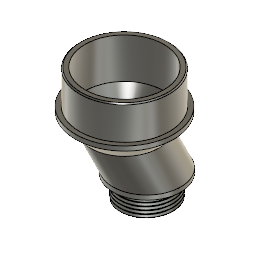
RobinairExhaustFilterAdapter (Autodesk Fusion 360 design; units mm, degrees)
Autodesk Fusion 360 part; units mm, degrees
sketch "Sketch1" plane through (0, 0, 0) normal (0, 1, 0) x (1, 0, 0)
  line L0 (0.0002, -40) -> (0.0002, 25) construction
  line L1 (-19.9998, -5.8576) -> (-19.9998, -20.8576)
  line L2 (-19.9998, -5.8576) -> (-21.9998, -5.8576)
  line L3 (-21.9998, -5.8576) -> (-21.9998, -3.8576)
  line L4 (-12.7498, 5.3924) -> (-11.7498, 5.3924)
  line L5 (-21.9998, -3.8576) -> (-12.7498, 5.3924)
  line L6 (-17.5998, -2.8517) -> (-17.5998, -20.8576)
  line L7 (-17.5998, 2.9924) -> (-8.9498, 2.9924)
  line L8 (-17.5998, -2.8517) -> (-17.5998, 2.9924)
  line L9 (-19.9998, -20.8576) -> (-17.5998, -20.8576)
  line L10 (-11.7557, 2.9924) -> (-17.5998, -2.8517)
  line L11 (-11.7498, 6.3924) -> (-8.9498, 6.3924)
  line L12 (-8.9498, 2.9924) -> (-8.9498, 6.3924)
  line L13 (-11.7498, 5.3924) -> (-11.7498, 6.3924)
  dimension "d1" = 15
  dimension "d2" = 20
  dimension "d3" = 2
  dimension "d4" = 2
  dimension "d7" = 45
  dimension "d14" = 2.4
  dimension "d15" = 45
  dimension "d16" = 2.4
  dimension "d17" = 2.4
  dimension "d19" = 1
  dimension "d20" = 11.75
  dimension "d21" = 2.8
  dimension "d30" = 1
  measures "d2" distance of L0 L1
  measures "d7" angle of L4 L5
  measures "d15" angle of L7 L10
  measures "d16" distance of L5 L10
  measures "d17" distance of L4 L7
  measures "d20" distance of L0 L13
revolve "Revolve1" add sketch "Sketch1" angle 360 about axis through (0.0002, 0, 40) along (0, 0, -1) contours L1 L2 L3 L5 L6 L8 L9 | L5 L7 L8 L10
chamfer "Chamfer1" distance 0.5 angle 45 1 edges at (-18.6463, 7.2323, 20.8576)
sketch "Sketch4" plane through (0, 0, 0) normal (0, 1, 0) x (1, 0, 0)
  line L0 (11.7561, 2.9924) -> (-11.7557, 2.9924)
  line L1 (0.0002, 2.9924) -> (0.0002, 28.4999) construction
  line L2 (10.0002, 2.9924) -> (10.0002, 28) construction
  line L3 (0.0002, 2.9924) -> (10.0002, 12.9924)
  line L4 (0.0002, 2.9924) -> (13.1671, 2.9924) construction
  dimension "d31" = 10
  dimension "d32" = 45
  measures "d31" distance of L1 L2
  measures "d32" angle of L3 L4
sweep "Sweep2" add 1 faces at (-13.9183, -1.3367, -2.9924) path "Sketch4" along L3
sketch "Sketch5" plane through (0, 0, -12.9924) normal (0, 0, -1) x (1, 0, 0)
  circle A0 centre (10.0002, 0) radius 15.15
  circle A1 centre (10.0002, 0) radius 11.7559
  circle A2 centre (10.0002, 0) radius 9.3559
  dimension "d40" = 2.4
extrude "Extrude1" add sketch "Sketch5" along normal blind 2 contours A0 | A1
sketch "Sketch6" plane through (0, 0, -14.9924) normal (0, 0, -1) x (1, 0, 0)
  circle A0 centre (10.0002, 0) radius 9.3559
  circle A1 centre (10.0002, 0) radius 15.15
  circle A2 centre (10.0002, 0) radius 11.75
  dimension "d44" = 23.5
  measures "d44" diameter of A2
extrude "Extrude2" add sketch "Sketch6" along normal blind 9.25 contours A2
thread "Thread3" "ISO Metric profile 24.0 M24x1.5 6g" major diameter 23.85 minor diameter 22.1319 pitch 1.5 angle 60 modelled right hand crest width 0.1875 on face at (21.6918, 1.1699, -18.0758) crest through (21.9252, 0, -14.8987)
chamfer "Chamfer3" distance 2.4 angle 45 1 edges at (1.2775, -3.3832, -12.9924)
equation "d44 = ( 11.75 * 2 ) * 1 mm"
